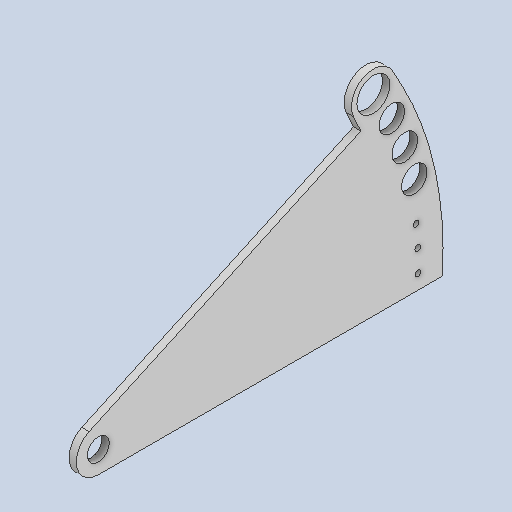
# Autodesk Inventor part: Shooter Side
Saved by Autodesk Inventor 2023 (Build 270158000, 158)
## iProperties
Created: 2023-11-15
Part Number: Shooter Side
Material: Generic
Document SubType Name: Modeling
Designer: jackc
Density: 1 g/cm^3
Appearance: Default
Author: jackc
Autodesk Inventor part; units mm, degrees
ref_plane "YZ Plane" through (0, 0, 0) normal (1, 0, 0) x (0, 1, 0)
ref_plane "XZ Plane" through (0, 0, 0) normal (0, 1, 0) x (-1, 0, 0)
ref_plane "XY Plane" through (0, 0, 0) normal (0, 0, 1) x (1, 0, 0)
sketch "Sketch1" plane through (0, 0, 0) normal (1, 0, 0) x (0, 1, 0)
  circle A0 centre (0, 0) radius 9.525
  arc A1 (-25.1608, -265.5105) -> (128.0642, -233.9411) centre (0, 0) ccw construction
  arc A2 (17.3208, 7.9305) -> (-19.05, 0) centre (0, 0) ccw
  line L0 (-19.05, 0) -> (-19.05, -297.8414)
  circle A3 centre (121.0878, -254.0152) radius 14.7 construction
  circle A4 centre (93.9242, -265.2625) radius 14.7 construction
  circle A5 centre (65.7355, -273.6143) radius 14.7 construction
  circle A6 centre (121.0878, -254.0152) radius 11.1125
  circle A7 centre (93.9242, -265.2625) radius 11.1125
  circle A8 centre (65.7355, -273.6143) radius 11.1125
  circle A9 centre (121.0878, -254.0152) radius 12.7 construction
  circle A10 centre (93.9242, -265.2625) radius 12.7 construction
  circle A11 centre (65.7355, -273.6143) radius 12.7 construction
  line L1 (17.3208, 7.9305) -> (125.0203, -227.293)
  arc A12 (-19.05, -276.2038) -> (132.3042, -243.2017) centre (0, 0) ccw construction
  arc A13 (-19.05, -297.8414) -> (141.312, -262.8751) centre (0, 0) ccw
  circle A14 centre (31.6741, -275.0422) radius 2.4892
  circle A15 centre (12.6854, -276.5692) radius 2.4892
  circle A16 centre (-6.3634, -276.7869) radius 2.4892
  arc A17 (-19.05, -286.3871) -> (136.5435, -252.4606) centre (0, 0) ccw construction
  line L2 (0, 0) -> (8.0964, -266.5771) construction
  line L3 (8.4048, -276.7324) -> (8.7133, -286.8877) construction
  line L4 (8.4048, -276.7324) -> (8.0964, -266.5771) construction
  line L5 (51.0397, -273.9694) -> (31.6741, -275.0422) construction
  line L6 (48.6698, -262.2215) -> (54.4639, -293.4384) construction
  line L7 (48.6698, -262.2215) -> (0, 0) construction
  circle A18 centre (147.1034, -238.1338) radius 14.2875
  arc A19 (156.1233, -254.9131) -> (139.1729, -220.813) centre (147.1034, -238.1338) ccw
  line L8 (139.1729, -220.813) -> (125.0203, -227.293)
  line L9 (128.0642, -233.9411) -> (141.312, -262.8751) construction
  line L10 (125.0203, -227.293) -> (128.0642, -233.9411) construction
  line L11 (156.1233, -254.9131) -> (141.312, -262.8751)
  dimension "d0" = 19.05
  dimension "d1" = 266.7
  dimension "d3" = 22.225
  dimension "d4" = 25.4
  dimension "d5" = 2
  dimension "d8" = 9.525
  dimension "d10" = 31.75
  dimension "d11" = 4.9784
  dimension "d12" = 19.05
  dimension "d13" = 19.05
  dimension "d14" = 12.7
  dimension "d17" = 287.02
  dimension "d19" = 19.05
  dimension "d20" = 28.575
  dimension "d22" = 4.7625
  dimension "d24" = 30.48
  constraints: 24 end point, 22 point on circle, 19 centre point, 10 tangent, 8 equal radius, 7 coincident, 6 concentric, 6 point on line, 5 collinear, 2 perpendicular, 1 vertical, 7 other
  measures "d0" diameter of A0
  measures "d1" radius of A1
  measures "d3" diameter of A8
  measures "d4" diameter of A9
  measures "d5" radial gap between concentric circles of A3 A9
  measures "d8" radial gap between concentric circles of A0 A2
  measures "d10" radial gap between concentric circles of A13 A1
  measures "d11" diameter of A16
  measures "d12" distance of A16.centre A15.centre
  measures "d13" distance of A15.centre L5.end
  measures "d14" distance of A12.start A16.centre
  measures "d17" radius of A17
  measures "d19" distance from line of L5.end L6
  measures "d20" diameter of A18
  measures "d22" radial gap between concentric circles of A19 A18
  measures "d24" distance of A18.centre A3.centre
extrude "Extrusion1" add sketch "Sketch1" along normal blind 6.35
equation "\"d1\" = BallSize + 0.5 * WheelSize - Compression"
equation "\"BallSize\" = 228.6"
equation "\"WheelSize\" = 101.6"
equation "\"Compression\" = 12.7"
body "Solid1"
